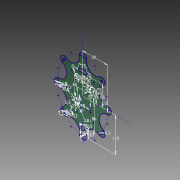
# Autodesk Inventor part: BodyTop
Saved by Autodesk Inventor 2015 SP2 (Build 190223200, 223)
## iProperties
Created: 2015-10-10
Part Number: BodyTop
Material: Generic
Document SubType Name: Modeling
Designer: styku
Density: 1 g/cm^3
Appearance: Clear - Green 1
Mass: 66.029 g
Surface Area: 479.519 cm^2
Volume: 66.029 cm^3
Author: styku
Autodesk Inventor part; units mm, degrees
ref_plane "YZ Plane" through (0, 0, 0) normal (1, 0, 0) x (0, 1, 0)
ref_plane "XZ Plane" through (0, 0, 0) normal (0, 1, 0) x (-1, 0, 0)
ref_plane "XY Plane" through (0, 0, 0) normal (0, 0, 1) x (1, 0, 0)
sketch "Sketch1" plane through (0, 0, 0) normal (0, 1, 0) x (-1, 0, 0)
  line L0 (0, -135) -> (0, 190) construction
  line L1 (111, 0) -> (-155, 0) construction
  ellipse E0 centre (0, 0) end of major axis (0, 110) minor radius 80 construction
  arc A0 (79.5622, -11.4917) -> (91.5, 0) centre (80, 0) ccw
  arc A1 (0, -121.5) -> (11.4442, -108.8687) centre (0, -110) ccw
  arc A2 (53.6974, -81.5386) -> (66.0076, -62.1493) centre (60.3721, -72.1738) ccw
  arc A3 (79.5622, -11.4917) -> (66.0076, -62.1493) centre (79.2711, -38.556) ccw
  arc A4 (53.6974, -81.5386) -> (11.4442, -108.8687) centre (37.9882, -103.5791) ccw
  arc A5 (-91.5, 0) -> (-79.5622, -11.4917) centre (-80, 0) ccw
  arc A6 (-11.4442, -108.8687) -> (0, -121.5) centre (0, -110) ccw
  arc A7 (-66.0076, -62.1493) -> (-53.6974, -81.5386) centre (-60.3721, -72.1738) ccw
  arc A8 (-66.0076, -62.1493) -> (-79.5622, -11.4917) centre (-79.2711, -38.556) ccw
  arc A9 (-11.4442, -108.8687) -> (-53.6974, -81.5386) centre (-37.9882, -103.5791) ccw
  arc A10 (91.5, 0) -> (79.5622, 11.4917) centre (80, 0) ccw
  arc A11 (11.4442, 108.8687) -> (0, 121.5) centre (0, 110) ccw
  arc A12 (66.0076, 62.1493) -> (53.6974, 81.5386) centre (60.3721, 72.1738) ccw
  arc A13 (66.0076, 62.1493) -> (79.5622, 11.4917) centre (79.2711, 38.556) ccw
  arc A14 (11.4442, 108.8687) -> (53.6974, 81.5386) centre (37.9882, 103.5791) ccw
  arc A15 (0, 121.5) -> (-11.4442, 108.8687) centre (0, 110) ccw
  arc A16 (-53.6974, 81.5386) -> (-11.4442, 108.8687) centre (-37.9882, 103.5791) ccw
  arc A17 (-53.6974, 81.5386) -> (-66.0076, 62.1493) centre (-60.3721, 72.1738) ccw
  arc A18 (-79.5622, 11.4917) -> (-66.0076, 62.1493) centre (-79.2711, 38.556) ccw
  arc A19 (-79.5622, 11.4917) -> (-91.5, 0) centre (-80, 0) ccw
  line L2 (53.0109, -83.8154) -> (69.937, -57.0473) construction
  circle A20 centre (56.3638, -78.5129) radius 0.5
  line L3 (66.5644, -76.0894) -> (34.2267, -55.6415) construction
  circle A21 centre (64.3804, -65.8348) radius 0.5
  line L4 (80, -8.2711) -> (80, 9) construction
  circle A22 centre (80, -7.5) radius 0.5
  line L5 (9.0844, -110) -> (-9.2812, -110) construction
  circle A23 centre (7.5, -110) radius 0.5
  circle A24 centre (-56.3638, -78.5129) radius 0.5
  circle A25 centre (-64.3804, -65.8348) radius 0.5
  circle A26 centre (-80, -7.5) radius 0.5
  circle A27 centre (-7.5, -110) radius 0.5
  circle A28 centre (56.3638, 78.5129) radius 0.5
  circle A29 centre (64.3804, 65.8348) radius 0.5
  circle A30 centre (80, 7.5) radius 0.5
  circle A31 centre (7.5, 110) radius 0.5
  circle A32 centre (-7.5, 110) radius 0.5
  circle A33 centre (-56.3638, 78.5129) radius 0.5
  circle A34 centre (-64.3804, 65.8348) radius 0.5
  circle A35 centre (-80, 7.5) radius 0.5
  circle A36 centre (10, -37) radius 1.905
  circle A37 centre (-15.6, 17.6) radius 1.905
  circle A38 centre (60.3721, -72.1738) radius 3.25
  circle A39 centre (0, -110) radius 3.25
  circle A40 centre (-60.3721, -72.1738) radius 3.25
  circle A41 centre (80, 0) radius 3.25
  circle A42 centre (-80, 0) radius 3.25
  circle A43 centre (60.3721, 72.1738) radius 3.25
  circle A44 centre (0, 110) radius 3.25
  circle A45 centre (-60.3721, 72.1738) radius 3.25
  circle A46 centre (-25, 32.5) radius 1.5
  circle A47 centre (-25, -32.5) radius 1.5
  circle A48 centre (25, 32.5) radius 1.5
  circle A49 centre (25, -32.5) radius 1.5
  line L6 (12.5, 65) -> (-12.5, 65)
  line L7 (-12.5, 65) -> (-12.5, 74)
  line L8 (-12.5, 74) -> (12.5, 74)
  line L9 (12.5, 74) -> (12.5, 65)
  line L10 (6, -95) -> (-6, -95)
  line L11 (-6, -95) -> (-6, -86)
  line L12 (-6, -86) -> (6, -86)
  line L13 (6, -86) -> (6, -95)
  circle A50 centre (50, 0) radius 1.75
  circle A51 centre (35.016, -56.1406) radius 1.75
  circle A52 centre (0, -80) radius 1.75
  circle A53 centre (-50, 0) radius 1.75
  circle A54 centre (-35.016, -56.1406) radius 1.75
  circle A55 centre (35.016, 56.1406) radius 1.75
  circle A56 centre (0, 80) radius 1.75
  circle A57 centre (-35.016, 56.1406) radius 1.75
  circle A58 centre (-24.5, 39) radius 1.375
  circle A59 centre (24.5, 39) radius 1.375
  circle A60 centre (-24.5, -19) radius 1.375
  circle A61 centre (24.5, -19) radius 1.375
  circle A62 centre (25, 52.5) radius 1.5
  circle A63 centre (-25, 52.5) radius 1.5
  circle A64 centre (25, -12.5) radius 1.5
  circle A65 centre (-25, -12.5) radius 1.5
  circle A66 centre (22.5, -26) radius 1.5
  circle A67 centre (-22.5, -26) radius 1.5
  circle A68 centre (22.5, -53.5) radius 1.5
  circle A69 centre (-22.5, -53.5) radius 1.5
  dimension "d0" = 110
  dimension "d1" = 80
  dimension "d2" = 23
  dimension "d3" = 23
  dimension "d4" = 23
  dimension "d6" = 1
  dimension "d7" = 7.5
  dimension "d8" = 1
  dimension "d9" = 7.5
  dimension "d12" = 1
  dimension "d13" = 7.5
  dimension "d16" = 3.81
  dimension "d17" = 3.81
  dimension "d18" = 10
  dimension "d19" = 37
  dimension "d21" = 15.6
  dimension "d22" = 6.5
  dimension "d23" = 6.5
  dimension "d24" = 6.5
  dimension "d25" = 6.5
  dimension "d26" = 6.5
  dimension "d29" = 3
  dimension "d30" = 25
  dimension "d31" = 32.5
  dimension "d34" = 9
  dimension "d35" = 25
  dimension "d36" = 65
  dimension "d40" = 54.6
  dimension "d41" = 12
  dimension "d42" = 9
  dimension "d43" = 86
  dimension "d47" = 3.5
  dimension "d48" = 30
  dimension "d49" = 3.5
  dimension "d50" = 30
  dimension "d51" = 3.5
  dimension "d52" = 30
  dimension "d61" = 2.75
  dimension "d62" = 24.5
  dimension "d63" = 39
  dimension "d66" = 49
  dimension "d69" = 58
  dimension "d74" = 3
  dimension "d75" = 20
  dimension "d76" = 0
  dimension "d79" = 50
  dimension "d82" = 65
  dimension "d85" = 3
  dimension "d88" = 45
  dimension "d91" = 27.5
  dimension "d94" = 26
  constraints: 70 centre point, 49 symmetric about line, 40 point on circle, 28 end point, 14 point on line, 8 horizontal, 7 vertical, 6 coincident, 4 parallel, 3 perpendicular, 2 tangent, 1 equal radius, 70 other
  measures "d2" diameter of A0
  measures "d3" diameter of A1
  measures "d4" diameter of A2
  measures "d6" diameter of A20
  measures "d7" distance from line of L3 A20.centre
  measures "d8" diameter of A22
  measures "d9" distance from line of L1 A22.centre
  measures "d12" diameter of A23
  measures "d13" distance from line of L0 A23.centre
  measures "d16" diameter of A36
  measures "d17" diameter of A37
  measures "d18" distance from line of L0 A36.centre
  measures "d19" distance from line of L1 A36.centre
  measures "d21" distance from line of L0 A37.centre
  measures "d22" diameter of A38
  measures "d23" diameter of A39
  measures "d24" diameter of A40
  measures "d25" diameter of A41
  measures "d26" diameter of A42
  measures "d29" diameter of A46
  measures "d30" distance from line of L0 A46.centre
  measures "d31" distance from line of A46.centre L1
  measures "d34" distance between parallel lines of L8 L6
  measures "d35" distance between parallel lines of L7 L9
  measures "d36" distance between parallel lines of L1 L6
  measures "d40" vertical distance of A37.centre A36.centre
  measures "d41" distance of L10.start L10.end
  measures "d42" distance between parallel lines of L12 L10
  measures "d43" distance between parallel lines of L1 L12
  measures "d47" diameter of A50
  measures "d48" distance of A0.centre A50.centre
  measures "d49" diameter of A51
  measures "d50" distance from line of L2 A51.centre
  measures "d51" diameter of A52
  measures "d52" distance of A1.centre A52.centre
  measures "d61" diameter of A58
  measures "d62" distance from line of L0 A58.centre
  measures "d63" distance from line of L1 A58.centre
  measures "d66" distance of A58.centre A59.centre
  measures "d69" distance of A58.centre A60.centre
  measures "d74" diameter of A62
  measures "d75" distance of A48.centre A62.centre
  measures "d76" horizontal distance of A62.centre A48.centre
  measures "d79" distance of A62.centre A63.centre
  measures "d82" distance of A62.centre A64.centre
  measures "d85" diameter of A66
  measures "d88" distance of A66.centre A67.centre
  measures "d91" distance of A66.centre A68.centre
  measures "d94" distance from line of L1 A66.centre
extrude "Extrusion2" add sketch "Sketch1" along normal blind 3 contours A3 A2 A4 A1 A6 A9 A7 A8 A5 A19 A18 A17 A16 A15 A11 A14 A12 A13 A10 A0 | A46 | A47 | A48 | A49 | L6 L7 L8 L9 | L10 L11 L12 L13 | A50 | A51 | A52 | A53 | A54 | A55 | A56 | A57 | A58 | A59 | A60 | A61 | A62 | A63 | A64 | A65 | A66 | A67 | A68 | A69
extrude "Extrusion3" cut sketch "Sketch1" along normal blind 11 contours A46 | A47 | A48 | A49
extrude "Extrusion4" cut sketch "Sketch1" along normal blind 10 contours L6 L7 L8 L9
extrude "Extrusion5" cut sketch "Sketch1" along normal blind 10 contours L10 L11 L12 L13
fillet "Fillet1" radius 2 8 edges at (-6, 1.5, -95) (6, 1.5, -95) (-6, 1.5, -86) (6, 1.5, -86) (-12.5, 1.5, 65) (12.5, 1.5, 65) (-12.5, 1.5, 74) (12.5, 1.5, 74)
extrude "Extrusion6" cut sketch "Sketch1" along normal blind 10 contours A50 | A51 | A52 | A53 | A54 | A55 | A56 | A57
sketch "Sketch2" plane through (0, 0, 0) normal (0, -1, 0) x (1, 0, 0)
  line L0 (-40, -16.5) -> (-37, -16.5)
  line L1 (-37, -16.5) -> (-37, -42.5)
  line L2 (-37, -42.5) -> (-40, -42.5)
  line L3 (-40, -42.5) -> (-40, -16.5)
  circle A0 centre (-25, -32.5) radius 1.5 projected
  line L4 (0, 18) -> (0, -62) construction
  line L5 (40, -16.5) -> (37, -16.5)
  line L6 (37, -16.5) -> (37, -42.5)
  line L7 (37, -42.5) -> (40, -42.5)
  line L8 (40, -42.5) -> (40, -16.5)
  line L9 (-42, 0) -> (57, 0) construction
  line L10 (-40, 16.5) -> (-37, 16.5)
  line L11 (-37, 16.5) -> (-37, 42.5)
  line L12 (-37, 42.5) -> (-40, 42.5)
  line L13 (-40, 42.5) -> (-40, 16.5)
  line L14 (40, 16.5) -> (37, 16.5)
  line L15 (37, 16.5) -> (37, 42.5)
  line L16 (37, 42.5) -> (40, 42.5)
  line L17 (40, 42.5) -> (40, 16.5)
  point P0 (0, 0)
  dimension "d55" = 12
  dimension "d56" = 3
  dimension "d57" = 26
  dimension "d58" = 16
  constraints: 36 end point, 12 symmetric about line, 3 horizontal, 2 parallel, 2 vertical, 1 perpendicular
  measures "d55" distance from line of A0.centre L1
  measures "d56" distance of L0.end L0.start
  measures "d57" distance between parallel lines of L2 L0
  measures "d58" distance from line of A0.centre L0
extrude "Extrusion7" cut sketch "Sketch2" against normal blind 33.25 contours L0 L1 L2 L3 | L8 L7 L6 L5 | L13 L12 L11 L10 | L14 L15 L16 L17
extrude "Extrusion8" cut sketch "Sketch1" along normal blind 10 contours A58 | A59 | A60 | A61
extrude "Extrusion9" cut sketch "Sketch1" along normal blind 10 contours A62 | A63 | A64 | A65 | A66 | A67 | A68 | A69
body "Solid2"
